Autodesk Fusion 360 part; units mm, degrees
(part 4 of 4)
  constraint vertical L5
  constraint horizontal L6
  constraint vertical L7
  constraint coincident L0.end L1.start
  constraint coincident L2.end L3.start
extrude "Extrude2" add sketch "Sketch3" along normal blind 0.36 separate body contours S0 S1 S2 S3 | S4 S5 S6 S7 | S8 S9 S10 S11 | S12 S13 S14 S15 | S16 S17 S18 S19 | S20 S21 S22 S23 | S24 S25 S26 S27 | S28 S29 S30 S31 | S32 S33 S34 S35 | S36 S37 S38 S39 | S40 S41 S42 S43 | S44 S45 S46 S47 | S48 S49 S50 S51 | S52 S53 S54 S55 | S56 S57 S58 S59 | S60 S61 S62 S63 | S64 S65 S66 S67 | S68 S69 S70 S71 | S72 S73 S74 S75 | S76 S77 S78 S79 | S80 S81 S82 S83 | S84 S85 S86 S87 | S88 S89 S90 S91 | S92 S93 S94 S95 | S96 S97 S98 S99 | S100 S101 S102 S103 | S104 S105 S106 S107 | S108 S109 S110 S111 | S112 S113 S114 S115 | S116 S117 S118 S119 | S120 S121 S122 S123 | S124 S125 S126 S127 | S128 S129 S130 S131 | S132 S133 S134 S135 | S136 S137 S138 S139 | S140 S141 S142 S143 | S144 S145 S146 S147 | S148 S149 S150 S151 | S152 S153 S154 S155 | S156 S157 S158 S159 | S160 S161 S162 S163 | S164 S165 S166 S167 | S168 S169 S170 S171 | S172 S173 S174 S175 | S176 S177 S178 S179 | S180 S181 S182 S183 | S184 S185 S186 S187 | S188 S189 S190 S191 | S192 S193 S194 S195 | S196 S197 S198 S199 | S200 S201 S202 S203 | S204 S205 S206 S207 | S208 S209 S210 S211 | S212 S213 S214 S215 | S216 S217 S218 S219 | S220 S221 S222 S223 | S224 S225 S226 S227 | S228 S229 S230 S231 | S232 S233 S234 S235 | S236 S237 S238 S239 | S240 S241 S242 S243 | S244 S245 S246 S247 | S248 S249 S250 S251 | S252 S253 S254 S255 | S256 S257 S258 S259 | S260 S261 S262 S263 | S264 S265 S266 S267 | S268 S269 S270 S271 | S272 S273 S274 S275 | S276 S277 S278 S279 | S280 S281 S282 S283 | S284 S285 S286 S287 | S288 S289 S290 S291 | S292 S293 S294 S295 | S296 S297 S298 S299 | S300 S301 S302 S303 | S304 S305 S306 S307 | S308 S309 S310 S311 | S312 S313 S314 S315 | S316 S317 S318 S319 | S320 S321 S322 S323 | S324 S325 S326 S327 | S328 S329 S330 S331 | S332 S333 S334 S335 | S336 S337 S338 S339 | S340 S341 S342 S343 | S344 S345 S346 S347 | S348 S349 S350 S351 | S352 S353 S354 S355 | S356 S357 S358 S359 | S360 S361 S362 S363 | S364 S365 S366 S367 | S368 S369 S370 S371 | S372 S373 S374 S375 | S376 S377 S378 S379 | S380 S381 S382 S383 | S384 S385 S386 S387 | S388 S389 S390 S391 | S392 S393 S394 S395 | S396 S397 S398 S399 | S400 S401 S402 S403 | S404 S405 S406 S407 | S408 S409 S410 S411 | S412 S413 S414 S415 | S416 S417 S418 S419 | S420 S421 S422 S423 | S424 S425 S426 S427 | S428 S429 S430 S431 | S432 S433 S434 S435 | S436 S437 S438 S439 | S440 S441 S442 S443 | S444 S445 S446 S447 | S448 S449 S450 S451 | S452 S453 S454 S455 | S456 S457 S458 S459 | S460 S461 S462 S463 | S464 S465 S466 S467 | S468 S469 S470 S471 | S472 S473 S474 S475 | S476 S477 S478 S479 | S480 S481 S482 S483 | S484 S485 S486 S487 | S488 S489 S490 S491 | S492 S493 S494 S495 | S496 S497 S498 S499 | S500 S501 S502 S503 | S504 S505 S506 S507 | S508 S509 S510 S511 | L0 L1 L2 L3 L4 L5 L6 L7 makes body 2
sketch "Sketch12" plane through (0, 0, 10.36) normal (0, 0, 1) x (-1, 0, 0)
  line L0 (1, 1) -> (-161, 1)
  line L1 (-161, 1) -> (-161, -81)
  line L2 (-161, -81) -> (1, -81)
  line L3 (1, -81) -> (1, 1)
  line L4 (-156, -79) -> (-4, -79)
  line L5 (-1, -76) -> (-1, -4)
  line L6 (-4, -1) -> (-156, -1)
  line L7 (-159, -4) -> (-159, -76)
  arc A0 (-1, -4) -> (-4, -1) centre (-4, -4) ccw
  arc A1 (-156, -1) -> (-159, -4) centre (-156, -4) ccw
  arc A2 (-159, -76) -> (-156, -79) centre (-156, -76) ccw
  arc A3 (-4, -79) -> (-1, -76) centre (-4, -76) ccw
  line L8 (-158, -88) -> (-2, -88)
  line L9 (8, -78) -> (8, -2)
  line L10 (-2, 8) -> (-158, 8)
  line L11 (-168, -2) -> (-168, -78)
  arc A4 (8, -2) -> (-2, 8) centre (-2, -2) ccw
  arc A5 (-2, -88) -> (8, -78) centre (-2, -78) ccw
  arc A6 (-158, 8) -> (-168, -2) centre (-158, -2) ccw
  arc A7 (-168, -78) -> (-158, -88) centre (-158, -78) ccw
  dimension "d63" = 82
  dimension "d64" = 162
  dimension "d66" = 3
  dimension "d67" = 3
  dimension "d69" = 10
  dimension "d134" = 7
  dimension "d135" = 7
  dimension "d136" = 7
  constraint horizontal L0
  constraint vertical L1
  constraint horizontal L2
  constraint vertical L3
  constraint tangent L5 A0
  constraint tangent L6 A0
  constraint tangent L6 A1
  constraint tangent L7 A1
  constraint tangent L4 A2
  constraint tangent L7 A2
  constraint equal A1 A2
  constraint tangent L4 A3
  constraint tangent L5 A3
  constraint equal A1 A3
  constraint tangent L9 A4
  constraint tangent L10 A4
  constraint tangent L8 A5
  constraint tangent L9 A5
  constraint equal A4 A5
  constraint tangent L10 A6
  constraint tangent L11 A6
  constraint equal A4 A6
  constraint tangent L8 A7
  constraint tangent L11 A7
  constraint equal A4 A7
  measures "d63" distance of L0.end L1.end
  measures "d64" distance of L0.start L0.end
  measures "d66" radius of A0
  measures "d67" radius of A1
  measures "d69" radius of A4
  measures "d134" distance of L3 L9
  measures "d135" distance of L0 L10
  measures "d136" distance of L1 L11
extrude "Extrude16" add sketch "Sketch12" along normal blind 2 separate body contours L0 L1 L2 L3 | L8 L9 L10 L11 A4 A5 A6 A7 makes body 3
sketch "Sketch13" plane through (0, 0, 10.36) normal (0, 0, -1) x (1, 0, 0)
  arc A0 (1, -76) -> (4, -79) centre (4, -76) ccw
  line L0 (1, -76) -> (1, -4)
  arc A1 (4, -1) -> (1, -4) centre (4, -4) ccw
  line L1 (4, -1) -> (156, -1)
  arc A2 (159, -4) -> (156, -1) centre (156, -4) ccw
  line L2 (159, -4) -> (159, -76)
  arc A3 (156, -79) -> (159, -76) centre (156, -76) ccw
  line L3 (156, -79) -> (4, -79)
  arc A4 (158, -88) -> (168, -78) centre (158, -78) ccw
  line L4 (168, -78) -> (168, -2)
  arc A5 (168, -2) -> (158, 8) centre (158, -2) ccw
  line L5 (158, 8) -> (2, 8)
  arc A6 (2, 8) -> (-8, -2) centre (2, -2) ccw
  line L6 (-8, -2) -> (-8, -78)
  arc A7 (-8, -78) -> (2, -88) centre (2, -78) ccw
  line L7 (2, -88) -> (158, -88)
  line L8 (-1, 1) -> (161, 1)
  line L9 (161, 1) -> (161, -81)
  line L10 (161, -81) -> (-1, -81)
  line L11 (-1, -81) -> (-1, 1)
  line L12 (-1, 1.2) -> (161, 1.2)
  dimension "d72" = -0.2
  constraint horizontal L8
  constraint vertical L9
  constraint horizontal L10
  constraint vertical L11
extrude "Extrude17" add sketch "Sketch13" along normal blind 15 separate body contours A4 L4 A5 L5 A6 L6 A7 L7 makes body 4
combine "Combine1" operation add target body 3 tool bodies 4
sketch "Sketch14" plane through (0, 0, 0) normal (0, 0, -1) x (1, 0, 0)
  line L0 (159, -78.4943) -> (151, -78.4943)
  line L1 (151, -78.4943) -> (151, -71.4943)
  line L2 (151, -71.4943) -> (159, -71.4943)
  line L3 (159, -71.4943) -> (159, -78.4943)
  line L4 (159, -68.4943) -> (151, -68.4943)
  line L5 (151, -68.4943) -> (151, -61.4943)
  line L6 (151, -61.4943) -> (159, -61.4943)
  line L7 (159, -61.4943) -> (159, -68.4943)
  line L8 (159, -58.4943) -> (151, -58.4943)
  line L9 (151, -58.4943) -> (151, -51.4943)
  line L10 (151, -51.4943) -> (159, -51.4943)
  line L11 (159, -51.4943) -> (159, -58.4943)
  line L12 (159, -48.4943) -> (151, -48.4943)
  line L13 (151, -48.4943) -> (151, -41.4943)
  line L14 (151, -41.4943) -> (159, -41.4943)
  line L15 (159, -41.4943) -> (159, -48.4943)
  line L16 (159, -38.4943) -> (151, -38.4943)
  line L17 (151, -38.4943) -> (151, -31.4943)
  line L18 (151, -31.4943) -> (159, -31.4943)
  line L19 (159, -31.4943) -> (159, -38.4943)
  line L20 (159, -28.4943) -> (151, -28.4943)
  line L21 (151, -28.4943) -> (151, -21.4943)
  line L22 (151, -21.4943) -> (159, -21.4943)
  line L23 (159, -21.4943) -> (159, -28.4943)
  line L24 (159, -18.4943) -> (151, -18.4943)
  line L25 (151, -18.4943) -> (151, -11.4943)
  line L26 (151, -11.4943) -> (159, -11.4943)
  line L27 (159, -11.4943) -> (159, -18.4943)
  line L28 (159, -8.4943) -> (151, -8.4943)
  line L29 (151, -8.4943) -> (151, -1.4943)
  line L30 (151, -1.4943) -> (159, -1.4943)
  line L31 (159, -1.4943) -> (159, -8.4943)
  line L32 (149, -78.4943) -> (141, -78.4943)
  line L33 (141, -78.4943) -> (141, -71.4943)
  line L34 (141, -71.4943) -> (149, -71.4943)
  line L35 (149, -71.4943) -> (149, -78.4943)
  line L36 (149, -68.4943) -> (141, -68.4943)
  line L37 (141, -68.4943) -> (141, -61.4943)
  line L38 (141, -61.4943) -> (149, -61.4943)
  line L39 (149, -61.4943) -> (149, -68.4943)
  line L40 (149, -58.4943) -> (141, -58.4943)
  line L41 (141, -58.4943) -> (141, -51.4943)
  line L42 (141, -51.4943) -> (149, -51.4943)
  line L43 (149, -51.4943) -> (149, -58.4943)
  line L44 (149, -48.4943) -> (141, -48.4943)
  line L45 (141, -48.4943) -> (141, -41.4943)
  line L46 (141, -41.4943) -> (149, -41.4943)
  line L47 (149, -41.4943) -> (149, -48.4943)
  line L48 (149, -38.4943) -> (141, -38.4943)
  line L49 (141, -38.4943) -> (141, -31.4943)
  line L50 (141, -31.4943) -> (149, -31.4943)
  line L51 (149, -31.4943) -> (149, -38.4943)
  line L52 (149, -28.4943) -> (141, -28.4943)
  line L53 (141, -28.4943) -> (141, -21.4943)
  line L54 (141, -21.4943) -> (149, -21.4943)
  line L55 (149, -21.4943) -> (149, -28.4943)
  line L56 (149, -18.4943) -> (141, -18.4943)
  line L57 (141, -18.4943) -> (141, -11.4943)
  line L58 (141, -11.4943) -> (149, -11.4943)
  line L59 (149, -11.4943) -> (149, -18.4943)
  line L60 (149, -8.4943) -> (141, -8.4943)
  line L61 (141, -8.4943) -> (141, -1.4943)
  line L62 (141, -1.4943) -> (149, -1.4943)
  line L63 (149, -1.4943) -> (149, -8.4943)
  line L64 (139, -78.4943) -> (131, -78.4943)
  line L65 (131, -78.4943) -> (131, -71.4943)
  line L66 (131, -71.4943) -> (139, -71.4943)
  line L67 (139, -71.4943) -> (139, -78.4943)
  line L68 (139, -68.4943) -> (131, -68.4943)
  line L69 (131, -68.4943) -> (131, -61.4943)
  line L70 (131, -61.4943) -> (139, -61.4943)
  line L71 (139, -61.4943) -> (139, -68.4943)
  line L72 (139, -58.4943) -> (131, -58.4943)
  line L73 (131, -58.4943) -> (131, -51.4943)
  line L74 (131, -51.4943) -> (139, -51.4943)
  line L75 (139, -51.4943) -> (139, -58.4943)
  line L76 (139, -48.4943) -> (131, -48.4943)
  line L77 (131, -48.4943) -> (131, -41.4943)
  line L78 (131, -41.4943) -> (139, -41.4943)
  line L79 (139, -41.4943) -> (139, -48.4943)
  line L80 (139, -38.4943) -> (131, -38.4943)
  line L81 (131, -38.4943) -> (131, -31.4943)
  line L82 (131, -31.4943) -> (139, -31.4943)
  line L83 (139, -31.4943) -> (139, -38.4943)
  line L84 (139, -28.4943) -> (131, -28.4943)
  line L85 (131, -28.4943) -> (131, -21.4943)
  line L86 (131, -21.4943) -> (139, -21.4943)
  line L87 (139, -21.4943) -> (139, -28.4943)
  line L88 (139, -18.4943) -> (131, -18.4943)
  line L89 (131, -18.4943) -> (131, -11.4943)
  line L90 (131, -11.4943) -> (139, -11.4943)
  line L91 (139, -11.4943) -> (139, -18.4943)
  line L92 (139, -8.4943) -> (131, -8.4943)
  line L93 (131, -8.4943) -> (131, -1.4943)
  line L94 (131, -1.4943) -> (139, -1.4943)
  line L95 (139, -1.4943) -> (139, -8.4943)
  line L96 (129, -78.4943) -> (121, -78.4943)
  line L97 (121, -78.4943) -> (121, -71.4943)
  line L98 (121, -71.4943) -> (129, -71.4943)
  line L99 (129, -71.4943) -> (129, -78.4943)
  line L100 (129, -68.4943) -> (121, -68.4943)
  line L101 (121, -68.4943) -> (121, -61.4943)
  line L102 (121, -61.4943) -> (129, -61.4943)
  line L103 (129, -61.4943) -> (129, -68.4943)
  line L104 (129, -58.4943) -> (121, -58.4943)
  line L105 (121, -58.4943) -> (121, -51.4943)
  line L106 (121, -51.4943) -> (129, -51.4943)
  line L107 (129, -51.4943) -> (129, -58.4943)
  line L108 (129, -48.4943) -> (121, -48.4943)
  line L109 (121, -48.4943) -> (121, -41.4943)
  line L110 (121, -41.4943) -> (129, -41.4943)
  line L111 (129, -41.4943) -> (129, -48.4943)
  line L112 (129, -38.4943) -> (121, -38.4943)
  line L113 (121, -38.4943) -> (121, -31.4943)
  line L114 (121, -31.4943) -> (129, -31.4943)
  line L115 (129, -31.4943) -> (129, -38.4943)
  line L116 (129, -28.4943) -> (121, -28.4943)
  line L117 (121, -28.4943) -> (121, -21.4943)
  line L118 (121, -21.4943) -> (129, -21.4943)
  line L119 (129, -21.4943) -> (129, -28.4943)
  line L120 (129, -18.4943) -> (121, -18.4943)
  line L121 (121, -18.4943) -> (121, -11.4943)
  line L122 (121, -11.4943) -> (129, -11.4943)
  line L123 (129, -11.4943) -> (129, -18.4943)
  line L124 (129, -8.4943) -> (121, -8.4943)
  line L125 (121, -8.4943) -> (121, -1.4943)
  line L126 (121, -1.4943) -> (129, -1.4943)
  line L127 (129, -1.4943) -> (129, -8.4943)
  line L128 (119, -78.4943) -> (111, -78.4943)
  line L129 (111, -78.4943) -> (111, -71.4943)
  line L130 (111, -71.4943) -> (119, -71.4943)
  line L131 (119, -71.4943) -> (119, -78.4943)
  line L132 (119, -68.4943) -> (111, -68.4943)
  line L133 (111, -68.4943) -> (111, -61.4943)
  line L134 (111, -61.4943) -> (119, -61.4943)
  line L135 (119, -61.4943) -> (119, -68.4943)
  line L136 (119, -58.4943) -> (111, -58.4943)
  line L137 (111, -58.4943) -> (111, -51.4943)
  line L138 (111, -51.4943) -> (119, -51.4943)
  line L139 (119, -51.4943) -> (119, -58.4943)
  line L140 (119, -48.4943) -> (111, -48.4943)
  line L141 (111, -48.4943) -> (111, -41.4943)
  line L142 (111, -41.4943) -> (119, -41.4943)
  line L143 (119, -41.4943) -> (119, -48.4943)
  line L144 (119, -38.4943) -> (111, -38.4943)
  line L145 (111, -38.4943) -> (111, -31.4943)
  line L146 (111, -31.4943) -> (119, -31.4943)
  line L147 (119, -31.4943) -> (119, -38.4943)
  line L148 (119, -28.4943) -> (111, -28.4943)
  line L149 (111, -28.4943) -> (111, -21.4943)
  line L150 (111, -21.4943) -> (119, -21.4943)
  line L151 (119, -21.4943) -> (119, -28.4943)
  line L152 (119, -18.4943) -> (111, -18.4943)
  line L153 (111, -18.4943) -> (111, -11.4943)
  line L154 (111, -11.4943) -> (119, -11.4943)
  line L155 (119, -11.4943) -> (119, -18.4943)
  line L156 (119, -8.4943) -> (111, -8.4943)
  line L157 (111, -8.4943) -> (111, -1.4943)
  line L158 (111, -1.4943) -> (119, -1.4943)
  line L159 (119, -1.4943) -> (119, -8.4943)
  line L160 (109, -78.4943) -> (101, -78.4943)
  line L161 (101, -78.4943) -> (101, -71.4943)
  line L162 (101, -71.4943) -> (109, -71.4943)
  line L163 (109, -71.4943) -> (109, -78.4943)
  line L164 (109, -68.4943) -> (101, -68.4943)
  line L165 (101, -68.4943) -> (101, -61.4943)
  line L166 (101, -61.4943) -> (109, -61.4943)
  line L167 (109, -61.4943) -> (109, -68.4943)
  line L168 (109, -58.4943) -> (101, -58.4943)
  line L169 (101, -58.4943) -> (101, -51.4943)
  line L170 (101, -51.4943) -> (109, -51.4943)
  line L171 (109, -51.4943) -> (109, -58.4943)
  line L172 (109, -48.4943) -> (101, -48.4943)
  line L173 (101, -48.4943) -> (101, -41.4943)
  line L174 (101, -41.4943) -> (109, -41.4943)
  line L175 (109, -41.4943) -> (109, -48.4943)
  line L176 (109, -38.4943) -> (101, -38.4943)
  line L177 (101, -38.4943) -> (101, -31.4943)
  line L178 (101, -31.4943) -> (109, -31.4943)
  line L179 (109, -31.4943) -> (109, -38.4943)
  line L180 (109, -28.4943) -> (101, -28.4943)
  line L181 (101, -28.4943) -> (101, -21.4943)
  line L182 (101, -21.4943) -> (109, -21.4943)
  line L183 (109, -21.4943) -> (109, -28.4943)
  line L184 (109, -18.4943) -> (101, -18.4943)
  line L185 (101, -18.4943) -> (101, -11.4943)
  line L186 (101, -11.4943) -> (109, -11.4943)
  line L187 (109, -11.4943) -> (109, -18.4943)
  line L188 (109, -8.4943) -> (101, -8.4943)
  line L189 (101, -8.4943) -> (101, -1.4943)
  line L190 (101, -1.4943) -> (109, -1.4943)
  line L191 (109, -1.4943) -> (109, -8.4943)
  line L192 (99, -78.4943) -> (91, -78.4943)
  line L193 (91, -78.4943) -> (91, -71.4943)
  line L194 (91, -71.4943) -> (99, -71.4943)
  line L195 (99, -71.4943) -> (99, -78.4943)
  line L196 (99, -68.4943) -> (91, -68.4943)
  line L197 (91, -68.4943) -> (91, -61.4943)
  line L198 (91, -61.4943) -> (99, -61.4943)
  line L199 (99, -61.4943) -> (99, -68.4943)
  line L200 (99, -58.4943) -> (91, -58.4943)
  line L201 (91, -58.4943) -> (91, -51.4943)
  line L202 (91, -51.4943) -> (99, -51.4943)
  line L203 (99, -51.4943) -> (99, -58.4943)
  line L204 (99, -48.4943) -> (91, -48.4943)
  line L205 (91, -48.4943) -> (91, -41.4943)
  line L206 (91, -41.4943) -> (99, -41.4943)
  line L207 (99, -41.4943) -> (99, -48.4943)
  line L208 (99, -38.4943) -> (91, -38.4943)
  line L209 (91, -38.4943) -> (91, -31.4943)
  line L210 (91, -31.4943) -> (99, -31.4943)
  line L211 (99, -31.4943) -> (99, -38.4943)
  line L212 (99, -28.4943) -> (91, -28.4943)
  line L213 (91, -28.4943) -> (91, -21.4943)
  line L214 (91, -21.4943) -> (99, -21.4943)
  line L215 (99, -21.4943) -> (99, -28.4943)
  line L216 (99, -18.4943) -> (91, -18.4943)
  line L217 (91, -18.4943) -> (91, -11.4943)
  line L218 (91, -11.4943) -> (99, -11.4943)
  line L219 (99, -11.4943) -> (99, -18.4943)
  line L220 (99, -8.4943) -> (91, -8.4943)
  line L221 (91, -8.4943) -> (91, -1.4943)
  line L222 (91, -1.4943) -> (99, -1.4943)
  line L223 (99, -1.4943) -> (99, -8.4943)
  line L224 (89, -78.4943) -> (81, -78.4943)
  line L225 (81, -78.4943) -> (81, -71.4943)
  line L226 (81, -71.4943) -> (89, -71.4943)
  line L227 (89, -71.4943) -> (89, -78.4943)
  line L228 (89, -68.4943) -> (81, -68.4943)
  line L229 (81, -68.4943) -> (81, -61.4943)
  line L230 (81, -61.4943) -> (89, -61.4943)
  line L231 (89, -61.4943) -> (89, -68.4943)
  line L232 (89, -58.4943) -> (81, -58.4943)
  line L233 (81, -58.4943) -> (81, -51.4943)
  line L234 (81, -51.4943) -> (89, -51.4943)
  line L235 (89, -51.4943) -> (89, -58.4943)
  line L236 (89, -48.4943) -> (81, -48.4943)
  line L237 (81, -48.4943) -> (81, -41.4943)
  line L238 (81, -41.4943) -> (89, -41.4943)
  line L239 (89, -41.4943) -> (89, -48.4943)
  line L240 (89, -38.4943) -> (81, -38.4943)
  line L241 (81, -38.4943) -> (81, -31.4943)
  line L242 (81, -31.4943) -> (89, -31.4943)
  line L243 (89, -31.4943) -> (89, -38.4943)
  line L244 (89, -28.4943) -> (81, -28.4943)
  line L245 (81, -28.4943) -> (81, -21.4943)
  line L246 (81, -21.4943) -> (89, -21.4943)
  line L247 (89, -21.4943) -> (89, -28.4943)
  line L248 (89, -18.4943) -> (81, -18.4943)
  line L249 (81, -18.4943) -> (81, -11.4943)
  line L250 (81, -11.4943) -> (89, -11.4943)
  line L251 (89, -11.4943) -> (89, -18.4943)
  line L252 (89, -8.4943) -> (81, -8.4943)
  line L253 (81, -8.4943) -> (81, -1.4943)
  line L254 (81, -1.4943) -> (89, -1.4943)
  line L255 (89, -1.4943) -> (89, -8.4943)
  line L256 (79, -78.4943) -> (71, -78.4943)
  line L257 (71, -78.4943) -> (71, -71.4943)
  line L258 (71, -71.4943) -> (79, -71.4943)
  line L259 (79, -71.4943) -> (79, -78.4943)
  line L260 (79, -68.4943) -> (71, -68.4943)
  line L261 (71, -68.4943) -> (71, -61.4943)
  line L262 (71, -61.4943) -> (79, -61.4943)
  line L263 (79, -61.4943) -> (79, -68.4943)
  line L264 (79, -58.4943) -> (71, -58.4943)
  line L265 (71, -58.4943) -> (71, -51.4943)
  line L266 (71, -51.4943) -> (79, -51.4943)
  line L267 (79, -51.4943) -> (79, -58.4943)
  line L268 (79, -48.4943) -> (71, -48.4943)
  line L269 (71, -48.4943) -> (71, -41.4943)
  line L270 (71, -41.4943) -> (79, -41.4943)
  line L271 (79, -41.4943) -> (79, -48.4943)
  line L272 (79, -38.4943) -> (71, -38.4943)
  line L273 (71, -38.4943) -> (71, -31.4943)
  line L274 (71, -31.4943) -> (79, -31.4943)
  line L275 (79, -31.4943) -> (79, -38.4943)
  line L276 (79, -28.4943) -> (71, -28.4943)
  line L277 (71, -28.4943) -> (71, -21.4943)
  line L278 (71, -21.4943) -> (79, -21.4943)
  line L279 (79, -21.4943) -> (79, -28.4943)
  line L280 (79, -18.4943) -> (71, -18.4943)
  line L281 (71, -18.4943) -> (71, -11.4943)
  line L282 (71, -11.4943) -> (79, -11.4943)
  line L283 (79, -11.4943) -> (79, -18.4943)
  line L284 (79, -8.4943) -> (71, -8.4943)
  line L285 (71, -8.4943) -> (71, -1.4943)
  line L286 (71, -1.4943) -> (79, -1.4943)
  line L287 (79, -1.4943) -> (79, -8.4943)
  line L288 (69, -78.4943) -> (61, -78.4943)
  line L289 (61, -78.4943) -> (61, -71.4943)
  line L290 (61, -71.4943) -> (69, -71.4943)
  line L291 (69, -71.4943) -> (69, -78.4943)
  line L292 (69, -68.4943) -> (61, -68.4943)
  line L293 (61, -68.4943) -> (61, -61.4943)
  line L294 (61, -61.4943) -> (69, -61.4943)
  line L295 (69, -61.4943) -> (69, -68.4943)
  line L296 (69, -58.4943) -> (61, -58.4943)
  line L297 (61, -58.4943) -> (61, -51.4943)
  line L298 (61, -51.4943) -> (69, -51.4943)
  line L299 (69, -51.4943) -> (69, -58.4943)
  line L300 (69, -48.4943) -> (61, -48.4943)
  line L301 (61, -48.4943) -> (61, -41.4943)
  line L302 (61, -41.4943) -> (69, -41.4943)
  line L303 (69, -41.4943) -> (69, -48.4943)
  line L304 (69, -38.4943) -> (61, -38.4943)
  line L305 (61, -38.4943) -> (61, -31.4943)
  line L306 (61, -31.4943) -> (69, -31.4943)
  line L307 (69, -31.4943) -> (69, -38.4943)
  line L308 (69, -28.4943) -> (61, -28.4943)
  line L309 (61, -28.4943) -> (61, -21.4943)
  line L310 (61, -21.4943) -> (69, -21.4943)
  line L311 (69, -21.4943) -> (69, -28.4943)
  line L312 (69, -18.4943) -> (61, -18.4943)
  line L313 (61, -18.4943) -> (61, -11.4943)
  line L314 (61, -11.4943) -> (69, -11.4943)
  line L315 (69, -11.4943) -> (69, -18.4943)
  line L316 (69, -8.4943) -> (61, -8.4943)
  line L317 (61, -8.4943) -> (61, -1.4943)
  line L318 (61, -1.4943) -> (69, -1.4943)
  line L319 (69, -1.4943) -> (69, -8.4943)
  line L320 (59, -78.4943) -> (51, -78.4943)
  line L321 (51, -78.4943) -> (51, -71.4943)
  line L322 (51, -71.4943) -> (59, -71.4943)
  line L323 (59, -71.4943) -> (59, -78.4943)
  line L324 (59, -68.4943) -> (51, -68.4943)
  line L325 (51, -68.4943) -> (51, -61.4943)
  line L326 (51, -61.4943) -> (59, -61.4943)
  line L327 (59, -61.4943) -> (59, -68.4943)
  line L328 (59, -58.4943) -> (51, -58.4943)
  line L329 (51, -58.4943) -> (51, -51.4943)
  line L330 (51, -51.4943) -> (59, -51.4943)
  line L331 (59, -51.4943) -> (59, -58.4943)
  line L332 (59, -48.4943) -> (51, -48.4943)
  line L333 (51, -48.4943) -> (51, -41.4943)
  line L334 (51, -41.4943) -> (59, -41.4943)
  line L335 (59, -41.4943) -> (59, -48.4943)
  line L336 (59, -38.4943) -> (51, -38.4943)
  line L337 (51, -38.4943) -> (51, -31.4943)
  line L338 (51, -31.4943) -> (59, -31.4943)
  line L339 (59, -31.4943) -> (59, -38.4943)
  line L340 (59, -28.4943) -> (51, -28.4943)
  line L341 (51, -28.4943) -> (51, -21.4943)
  line L342 (51, -21.4943) -> (59, -21.4943)
  line L343 (59, -21.4943) -> (59, -28.4943)
  line L344 (59, -18.4943) -> (51, -18.4943)
  line L345 (51, -18.4943) -> (51, -11.4943)
  line L346 (51, -11.4943) -> (59, -11.4943)
  line L347 (59, -11.4943) -> (59, -18.4943)
  line L348 (59, -8.4943) -> (51, -8.4943)
  line L349 (51, -8.4943) -> (51, -1.4943)
  line L350 (51, -1.4943) -> (59, -1.4943)
  line L351 (59, -1.4943) -> (59, -8.4943)
  line L352 (49, -78.4943) -> (41, -78.4943)
  line L353 (41, -78.4943) -> (41, -71.4943)
  line L354 (41, -71.4943) -> (49, -71.4943)
  line L355 (49, -71.4943) -> (49, -78.4943)
  line L356 (49, -68.4943) -> (41, -68.4943)
  line L357 (41, -68.4943) -> (41, -61.4943)
  line L358 (41, -61.4943) -> (49, -61.4943)
  line L359 (49, -61.4943) -> (49, -68.4943)
  line L360 (49, -58.4943) -> (41, -58.4943)
  line L361 (41, -58.4943) -> (41, -51.4943)
  line L362 (41, -51.4943) -> (49, -51.4943)
  line L363 (49, -51.4943) -> (49, -58.4943)
  line L364 (49, -48.4943) -> (41, -48.4943)
  line L365 (41, -48.4943) -> (41, -41.4943)
  line L366 (41, -41.4943) -> (49, -41.4943)
  line L367 (49, -41.4943) -> (49, -48.4943)
  line L368 (49, -38.4943) -> (41, -38.4943)
  line L369 (41, -38.4943) -> (41, -31.4943)
  line L370 (41, -31.4943) -> (49, -31.4943)
  line L371 (49, -31.4943) -> (49, -38.4943)
  line L372 (49, -28.4943) -> (41, -28.4943)
  line L373 (41, -28.4943) -> (41, -21.4943)
  line L374 (41, -21.4943) -> (49, -21.4943)
  line L375 (49, -21.4943) -> (49, -28.4943)
  line L376 (49, -18.4943) -> (41, -18.4943)
  line L377 (41, -18.4943) -> (41, -11.4943)
  line L378 (41, -11.4943) -> (49, -11.4943)
  line L379 (49, -11.4943) -> (49, -18.4943)
  line L380 (49, -8.4943) -> (41, -8.4943)
  line L381 (41, -8.4943) -> (41, -1.4943)
  line L382 (41, -1.4943) -> (49, -1.4943)
  line L383 (49, -1.4943) -> (49, -8.4943)
  line L384 (39, -78.4943) -> (31, -78.4943)
  line L385 (31, -78.4943) -> (31, -71.4943)
  line L386 (31, -71.4943) -> (39, -71.4943)
  line L387 (39, -71.4943) -> (39, -78.4943)
  line L388 (39, -68.4943) -> (31, -68.4943)
  line L389 (31, -68.4943) -> (31, -61.4943)
  line L390 (31, -61.4943) -> (39, -61.4943)
  line L391 (39, -61.4943) -> (39, -68.4943)
  line L392 (39, -58.4943) -> (31, -58.4943)
  line L393 (31, -58.4943) -> (31, -51.4943)
  line L394 (31, -51.4943) -> (39, -51.4943)
  line L395 (39, -51.4943) -> (39, -58.4943)
  line L396 (39, -48.4943) -> (31, -48.4943)
  line L397 (31, -48.4943) -> (31, -41.4943)
  line L398 (31, -41.4943) -> (39, -41.4943)
  line L399 (39, -41.4943) -> (39, -48.4943)
  line L400 (39, -38.4943) -> (31, -38.4943)
  line L401 (31, -38.4943) -> (31, -31.4943)
  line L402 (31, -31.4943) -> (39, -31.4943)
  line L403 (39, -31.4943) -> (39, -38.4943)
  line L404 (39, -28.4943) -> (31, -28.4943)
  line L405 (31, -28.4943) -> (31, -21.4943)
  line L406 (31, -21.4943) -> (39, -21.4943)
  line L407 (39, -21.4943) -> (39, -28.4943)
  line L408 (39, -18.4943) -> (31, -18.4943)
  line L409 (31, -18.4943) -> (31, -11.4943)
  line L410 (31, -11.4943) -> (39, -11.4943)
  line L411 (39, -11.4943) -> (39, -18.4943)
  line L412 (39, -8.4943) -> (31, -8.4943)
  line L413 (31, -8.4943) -> (31, -1.4943)
  line L414 (31, -1.4943) -> (39, -1.4943)
  line L415 (39, -1.4943) -> (39, -8.4943)
  line L416 (29, -78.4943) -> (21, -78.4943)
  line L417 (21, -78.4943) -> (21, -71.4943)
  line L418 (21, -71.4943) -> (29, -71.4943)
  line L419 (29, -71.4943) -> (29, -78.4943)
  line L420 (29, -68.4943) -> (21, -68.4943)
  line L421 (21, -68.4943) -> (21, -61.4943)
  line L422 (21, -61.4943) -> (29, -61.4943)
  line L423 (29, -61.4943) -> (29, -68.4943)
  line L424 (29, -58.4943) -> (21, -58.4943)
  line L425 (21, -58.4943) -> (21, -51.4943)
  line L426 (21, -51.4943) -> (29, -51.4943)
  line L427 (29, -51.4943) -> (29, -58.4943)
  line L428 (29, -48.4943) -> (21, -48.4943)
  line L429 (21, -48.4943) -> (21, -41.4943)
  line L430 (21, -41.4943) -> (29, -41.4943)
  line L431 (29, -41.4943) -> (29, -48.4943)
  line L432 (29, -38.4943) -> (21, -38.4943)
  line L433 (21, -38.4943) -> (21, -31.4943)
  line L434 (21, -31.4943) -> (29, -31.4943)
  line L435 (29, -31.4943) -> (29, -38.4943)
  line L436 (29, -28.4943) -> (21, -28.4943)
  line L437 (21, -28.4943) -> (21, -21.4943)
  line L438 (21, -21.4943) -> (29, -21.4943)
  line L439 (29, -21.4943) -> (29, -28.4943)
  line L440 (29, -18.4943) -> (21, -18.4943)
  line L441 (21, -18.4943) -> (21, -11.4943)
  line L442 (21, -11.4943) -> (29, -11.4943)
  line L443 (29, -11.4943) -> (29, -18.4943)
  line L444 (29, -8.4943) -> (21, -8.4943)
  line L445 (21, -8.4943) -> (21, -1.4943)
  line L446 (21, -1.4943) -> (29, -1.4943)
  line L447 (29, -1.4943) -> (29, -8.4943)
  line L448 (19, -78.4943) -> (11, -78.4943)
  line L449 (11, -78.4943) -> (11, -71.4943)
  line L450 (11, -71.4943) -> (19, -71.4943)
  line L451 (19, -71.4943) -> (19, -78.4943)
  line L452 (19, -68.4943) -> (11, -68.4943)
  line L453 (11, -68.4943) -> (11, -61.4943)
  line L454 (11, -61.4943) -> (19, -61.4943)
  line L455 (19, -61.4943) -> (19, -68.4943)
  line L456 (19, -58.4943) -> (11, -58.4943)
  line L457 (11, -58.4943) -> (11, -51.4943)
  line L458 (11, -51.4943) -> (19, -51.4943)
  line L459 (19, -51.4943) -> (19, -58.4943)
  line L460 (19, -48.4943) -> (11, -48.4943)
  line L461 (11, -48.4943) -> (11, -41.4943)
  line L462 (11, -41.4943) -> (19, -41.4943)
  line L463 (19, -41.4943) -> (19, -48.4943)
  line L464 (19, -38.4943) -> (11, -38.4943)
  line L465 (11, -38.4943) -> (11, -31.4943)
  line L466 (11, -31.4943) -> (19, -31.4943)
  line L467 (19, -31.4943) -> (19, -38.4943)
  line L468 (19, -28.4943) -> (11, -28.4943)
  line L469 (11, -28.4943) -> (11, -21.4943)
  line L470 (11, -21.4943) -> (19, -21.4943)
  line L471 (19, -21.4943) -> (19, -28.4943)
  line L472 (19, -18.4943) -> (11, -18.4943)
  line L473 (11, -18.4943) -> (11, -11.4943)
  line L474 (11, -11.4943) -> (19, -11.4943)
  line L475 (19, -11.4943) -> (19, -18.4943)
  line L476 (19, -8.4943) -> (11, -8.4943)
  line L477 (11, -8.4943) -> (11, -1.4943)
  line L478 (11, -1.4943) -> (19, -1.4943)
  line L479 (19, -1.4943) -> (19, -8.4943)
  line L480 (9, -78.4943) -> (1, -78.4943)
  line L481 (1, -78.4943) -> (1, -71.4943)
  line L482 (1, -71.4943) -> (9, -71.4943)
  line L483 (9, -71.4943) -> (9, -78.4943)
  line L484 (9, -68.4943) -> (1, -68.4943)
  line L485 (1, -68.4943) -> (1, -61.4943)
  line L486 (1, -61.4943) -> (9, -61.4943)
  line L487 (9, -61.4943) -> (9, -68.4943)
  line L488 (9, -58.4943) -> (1, -58.4943)
  line L489 (1, -58.4943) -> (1, -51.4943)
  line L490 (1, -51.4943) -> (9, -51.4943)
  line L491 (9, -51.4943) -> (9, -58.4943)
  line L492 (9, -48.4943) -> (1, -48.4943)
  line L493 (1, -48.4943) -> (1, -41.4943)
  line L494 (1, -41.4943) -> (9, -41.4943)
  line L495 (9, -41.4943) -> (9, -48.4943)
  line L496 (9, -38.4943) -> (1, -38.4943)
  line L497 (1, -38.4943) -> (1, -31.4943)
  line L498 (1, -31.4943) -> (9, -31.4943)
  line L499 (9, -31.4943) -> (9, -38.4943)
  line L500 (9, -28.4943) -> (1, -28.4943)
  line L501 (1, -28.4943) -> (1, -21.4943)
  line L502 (1, -21.4943) -> (9, -21.4943)
  line L503 (9, -21.4943) -> (9, -28.4943)
  line L504 (9, -18.4943) -> (1, -18.4943)
  line L505 (1, -18.4943) -> (1, -11.4943)
  line L506 (1, -11.4943) -> (9, -11.4943)
  line L507 (9, -11.4943) -> (9, -18.4943)
  line L508 (9, -8.4943) -> (1, -8.4943)
  line L509 (1, -8.4943) -> (1, -1.4943)
  line L510 (1, -1.4943) -> (9, -1.4943)
  line L511 (9, -1.4943) -> (9, -8.4943)
  line L512 (161, 1) -> (-1, 1)
  line L513 (-1, 1) -> (-1, -81)
  line L514 (-1, -81) -> (161, -81)
  line L515 (161, -81) -> (161, 1)
  line L516 (-1, 1) -> (161, 1)
  line L517 (161, 1) -> (161, -81)
  line L518 (161, -81) -> (-1, -81)
  line L519 (-1, -81) -> (-1, 1)
  line L520 (-0.5, -81) -> (-0.5, 0.5)
  line L521 (-0.5, 0.5) -> (161, 0.5)
  line L522 (-1, 1) -> (-1, -19)
  line L523 (-1, -19) -> (3, -19)
  line L524 (-1, -81) -> (-1, -61)
  line L525 (-1, -61) -> (3, -61)
  line L526 (6, -71) -> (6, -64)
  line L527 (6, -16) -> (6, -9)
  line L528 (75.1065, -9) -> (75.1065, -74)
  line L529 (79, -74) -> (80.1065, -74)
  line L530 (80.1065, -6) -> (79, -6)
  line L531 (75.1065, -6) -> (75.1065, -71)
  line L532 (83.1065, -37.5) -> (153.9065, -37.5)
  line L533 (153.9065, -42.5) -> (83.1065, -42.5)
  line L534 (153.9065, -37.5) -> (151, -37.5)
  line L535 (151, -42.5) -> (153.9065, -42.5)
  line L536 (80.1065, -71) -> (80.1065, -45.5)
  line L537 (80.1065, -34.5) -> (80.1065, -9)
  line L538 (154, -9) -> (154, -34.5)
  line L539 (154, -45.5) -> (154, -71)
  line L540 (151, -74) -> (83.1065, -74)
  line L541 (72.1065, -74) -> (9, -74)
  line L542 (9, -6) -> (72.1065, -6)
  line L543 (83.1065, -6) -> (151, -6)
  arc A0 (75.1065, -9) -> (72.1065, -6) centre (72.1065, -9) ccw
  arc A1 (83.1065, -6) -> (80.1065, -9) centre (83.1065, -9) ccw
  arc A2 (80.1065, -34.5) -> (83.1065, -37.5) centre (83.1065, -34.5) ccw
  arc A3 (83.1065, -42.5) -> (80.1065, -45.5) centre (83.1065, -45.5) ccw
  arc A4 (151, -37.5) -> (154, -34.5) centre (151, -34.5) ccw
  arc A5 (154, -9) -> (151, -6) centre (151, -9) ccw
  arc A6 (154, -45.5) -> (151, -42.5) centre (151, -45.5) ccw
  arc A7 (80.1065, -71) -> (83.1065, -74) centre (83.1065, -71) ccw
  arc A8 (151, -74) -> (154, -71) centre (151, -71) ccw
  arc A9 (72.1065, -74) -> (75.1065, -71) centre (72.1065, -71) ccw
  arc A10 (6, -71) -> (9, -74) centre (9, -71) ccw
  arc A11 (6, -64) -> (3, -61) centre (3, -64) ccw
  arc A12 (3, -19) -> (6, -16) centre (3, -16) ccw
  arc A13 (9, -6) -> (6, -9) centre (9, -9) ccw
  point P0 (80.1065, -37.5)
  point P1 (80.1065, -42.5)
  dimension "d75" = 0.5
  dimension "d77" = 20
  dimension "d78" = 5
  dimension "d80" = 73.8
  dimension "d81" = 5
  dimension "d82" = 3
  constraint horizontal L516
  constraint vertical L517
  constraint horizontal L518
  constraint vertical L519
  constraint coincident L514.end L515.start
  constraint coincident L512.end L513.start
  constraint perpendicular L512 L522
  constraint perpendicular L523 L526
  constraint coincident L513 L524.end
  constraint perpendicular L525 L526
  constraint collinear L526 L527
  constraint coincident L528.end L540
  constraint perpendicular L528 L540
  constraint horizontal L529
  constraint vertical L536
  constraint horizontal L530
  constraint vertical L531
  constraint coincident L530.start L542
  constraint horizontal L532
  constraint horizontal L533
  constraint horizontal L534
  constraint horizontal L535
  constraint collinear L536 L537
  constraint collinear L538 L539
  constraint coincident L259 L529.start
  constraint collinear L540 L541
  constraint coincident L287 L530.end
  constraint collinear L542 L543
  constraint tangent L528 A0
  constraint tangent L542 A0
  constraint coincident L530.start L537
  constraint tangent L543 A1
  constraint tangent L537 A1
  constraint equal A0 A1
  constraint coincident P0 L532
  constraint coincident P0 L537
  constraint tangent L532 A2
  constraint tangent L537 A2
  constraint equal A0 A2
  constraint coincident P1 L533
  constraint coincident P1 L536
  constraint tangent L533 A3
  constraint tangent L536 A3
  constraint equal A0 A3
  constraint tangent L534 A4
  constraint tangent L538 A4
  constraint equal A0 A4
  constraint tangent L538 A5
  constraint tangent L543 A5
  constraint equal A0 A5
  constraint tangent L535 A6
  constraint tangent L539 A6
  constraint equal A0 A6
  constraint coincident L529.start L540
  constraint coincident L529.end L536
  constraint tangent L540 A7
  constraint tangent L536 A7
  constraint equal A0 A7
  constraint tangent L539 A8
  constraint tangent L540 A8
  constraint equal A0 A8
  constraint coincident L528.end L531
  constraint tangent L541 A9
  constraint tangent L531 A9
  constraint equal A0 A9
  constraint tangent L526 A10
  constraint tangent L541 A10
  constraint equal A0 A10
  constraint tangent L525 A11
  constraint tangent L526 A11
  constraint equal A0 A11
  constraint tangent L523 A12
  constraint tangent L527 A12
  constraint equal A0 A12
  constraint tangent L527 A13
  constraint tangent L542 A13
  constraint equal A0 A13
  measures "d77" distance of L512.end L522.end
  measures "d78" distance of L528.end L529.end
  measures "d80" distance of P0 L532.end
  measures "d81" distance of P0 P1
  measures "d82" radius of A0
extrude "Extrude18" add sketch "Sketch14" along normal blind 4.64 separate body contours L0 L1 L2 L3 A8 | L32 L33 L35 L540 | L4 L6 L7 L539 | L64 L65 L67 L540 | L8 L10 L11 L539 | L96 L97 L99 L540 | L12 L13 L14 L15 L539 A6 | L128 L129 L131 L540 | L160 L161 L163 L540 | L45 L46 L47 L533 | L192 L193 L195 L540 | L77 L78 L79 L533 | L224 L225 L227 L540 A7 | L109 L110 L111 L533 | L141 L142 L143 L533 | L173 L174 L175 L533 | L237 L238 L239 L533 A3 | L205 L206 L207 L533 | L16 L17 L18 L19 L538 A4 | L48 L49 L51 L532 | L20 L22 L23 L538 | L80 L81 L83 L532 | L24 L26 L27 L538 | L112 L113 L115 L532 | L28 L29 L30 L31 A5 | L144 L145 L147 L532 | L61 L62 L63 L543 | L176 L177 L179 L532 | L93 L94 L95 L543 | L208 L209 L211 L532 | L125 L126 L127 L543 | L240 L241 L243 L532 A2 | L157 L158 L159 L543 | L189 L190 L191 L543 | L253 L254 L255 L543 A1 | L221 L222 L223 L543 | L256 L257 L258 L259 L260 L262 L263 L264 L266 L267 L268 L270 L271 L272 L274 L275 L276 L278 L279 L280 L282 L283 L284 L285 L286 L287 L288 L289 L291 L317 L318 L319 L320 L321 L323 L349 L350 L351 L352 L353 L355 L381 L382 L383 L384 L385 L387 L413 L414 L415 L416 L417 L419 L445 L446 L447 L448 L449 L451 L477 L478 L479 L480 L481 L482 L483 L484 L485 L486 L504 L505 L506 L508 L509 L510 L511 L514 L515 L517 L518 L520 L521 L523 L525 L526 L527 L528 L531 L541 L542 A10 A11 A12 A13 | L256 L257 L258 L259 L541 A9 | L288 L289 L291 L541 | L320 L321 L323 L541 | L260 L262 L263 L528 L531 | L352 L353 L355 L541 | L264 L266 L267 L528 L531 | L384 L385 L387 L541 | L268 L270 L271 L528 L531 | L416 L417 L419 L541 | L272 L274 L275 L528 L531 | L448 L449 L451 L541 | L276 L278 L279 L528 L531 | L480 L481 L482 L483 A10 | L280 L282 L283 L528 L531 | L484 L485 L486 L526 A11 | L284 L285 L286 L287 L542 A0 | L317 L318 L319 L542 | L349 L350 L351 L542 | L504 L505 L506 L527 A12 | L381 L382 L383 L542 | L413 L414 L415 L542 | L508 L509 L510 L511 A13 | L445 L446 L447 L542 | L477 L478 L479 L542 makes body 5
sketch "Sketch15" plane through (0, 0, -4.64) normal (0, 0, -1) x (1, 0, 0)
  line L0 (161, -81) -> (-1, -81)
  line L1 (-1, -81) -> (-1, 1)
  line L2 (-1, 1) -> (161, 1)
  line L3 (161, 1) -> (161, -81)
  line L4 (2, -88) -> (158, -88)
  arc A0 (158, -88) -> (168, -78) centre (158, -78) ccw
  line L5 (168, -78) -> (168, -2)
  arc A1 (168, -2) -> (158, 8) centre (158, -2) ccw
  line L6 (158, 8) -> (2, 8)
  arc A2 (2, 8) -> (-8, -2) centre (2, -2) ccw
  line L7 (-8, -2) -> (-8, -78)
  arc A3 (-8, -78) -> (2, -88) centre (2, -78) ccw
extrude "Extrude19" add sketch "Sketch15" along normal blind 7 separate body contours L0 L1 L2 L3 | L4 A0 L5 A1 L6 A2 L7 A3 makes body 6
combine "Combine2" operation add target body 5 tool bodies 6
sketch "Sketch16" plane through (0, 0, -4.64) normal (0, 0, 1) x (-1, 0, 0)
  arc A0 (-2, -88) -> (8, -78) centre (-2, -78) ccw
  line L0 (8, -78) -> (8, -2)
  arc A1 (8, -2) -> (-2, 8) centre (-2, -2) ccw
  line L1 (-2, 8) -> (-158, 8)
  arc A2 (-158, 8) -> (-168, -2) centre (-158, -2) ccw
  line L2 (-168, -2) -> (-168, -78)
  arc A3 (-168, -78) -> (-158, -88) centre (-158, -78) ccw
  line L3 (-158, -88) -> (-2, -88)
  line L4 (-75.0636, -8.4943) -> (-75.1065, -8.4943)
  line L5 (-75.1065, -8.4943) -> (-75.1065, -71.4943)
  line L6 (-75.1065, -71.4943) -> (-75.0655, -71.4943)
  arc A4 (-75.0655, -71.4943) -> (-72.1065, -74) centre (-72.1065, -71) ccw
  line L7 (-72.1065, -74) -> (-9, -74)
  arc A5 (-9, -74) -> (-6, -71) centre (-9, -71) ccw
  line L8 (-6, -71) -> (-6, -64)
  arc A6 (-3, -61) -> (-6, -64) centre (-3, -64) ccw
  line L9 (-3, -61) -> (0.5, -61)
  line L10 (0.5, -61) -> (0.5, -81)
  line L11 (0.5, -81) -> (-161, -81)
  line L12 (-161, -81) -> (-161, 0.5)
  line L13 (-161, 0.5) -> (0.5, 0.5)
  line L14 (0.5, 0.5) -> (0.5, -19)
  line L15 (0.5, -19) -> (-3, -19)
  arc A7 (-6, -16) -> (-3, -19) centre (-3, -16) ccw
  line L16 (-6, -16) -> (-6, -9)
  arc A8 (-6, -9) -> (-9, -6) centre (-9, -9) ccw
  line L17 (-9, -6) -> (-72.1065, -6)
  arc A9 (-72.1065, -6) -> (-75.0636, -8.4943) centre (-72.1065, -9) ccw
  line L18 (0.5, -81) -> (-161, -81)
  line L19 (-161, -81) -> (-161, 0.5)
  line L20 (-161, 0.5) -> (0.5, 0.5)
  line L21 (0.5, 0.5) -> (0.5, -81)
  line L22 (0.5, -61) -> (8, -61)
  line L23 (8, -61) -> (8, -18.999)
  line L24 (8, -18.999) -> (0.5, -18.999)
  line L25 (0.5, -18.999) -> (0.5, -61)
  line L26 (4.25, -18.999) -> (4.25, -61)
  line L27 (8.2113, -27.4995) -> (0.2887, -27.4995)
  line L28 (0.2887, -27.4995) -> (0.2887, -52.4995)
  line L29 (0.2887, -52.4995) -> (8.2113, -52.4995)
  line L30 (8.2113, -52.4995) -> (8.2113, -27.4995)
  line L31 (8.2113, -27.4995) -> (0.2887, -52.4995) construction
  line L32 (0.2887, -27.4995) -> (8.2113, -52.4995) construction
  point P0 (4.25, -39.9995)
  dimension "d89" = 25
  constraint horizontal L18
  constraint vertical L19
  constraint horizontal L20
  constraint vertical L21
  constraint coincident L12.end L13.start
  constraint coincident L10.end L11.start
  constraint horizontal L22
  constraint vertical L23
  constraint horizontal L24
  constraint vertical L25
  constraint coincident L0 L23.end
  constraint coincident L9.end L10.start
  constraint midpoint L24 L26.start
  constraint midpoint L22 L26.end
  constraint perpendicular L22 L26
  constraint horizontal L27
  constraint perpendicular L27 L28
  constraint parallel L27 L29
  constraint parallel L28 L30
  constraint coincident L31 P0
  constraint coincident L32 P0
  constraint midpoint L26 P0
  measures "d89" distance of L27.end L28.end
extrude "Extrude20" cut sketch "Sketch16" against normal blind 4 contours L4 L5 L6 A4 L7 A5 L8 A6 L9 L15 A7 L16 A8 L17 A9 L21 L25 L27 L28 L29 | L21 L25 L27 L28 L29 bodies 5
extrude "Extrude21" cut sketch "Sketch16" along normal blind 4.64 contours L0 L23 L26 L27 L29 | L21 L25 L26 L27 L29 bodies 3
fillet "Fillet1" radius 2 2 edges at (-4.5, 52.4995, 0) (-4.5, 27.4995, 0) on bodies 3
extrude "Extrude22" cut sketch "Sketch16" against normal blind 4 contours L0 L23 L26 L27 L29 | L21 L25 L26 L27 L29 bodies 5
fillet "Fillet2" radius 2 2 edges at (-4.25, 27.4995, -8.64) (-4.25, 52.4995, -8.64) on bodies 5
fillet "Fillet4" radius 2 8 edges at (80, -8, 12.36) (165.0711, -5.0711, 12.36) (168, 40, 12.36) (165.0711, 85.0711, 12.36) (80, 88, 12.36) (-5.0711, 85.0711, 12.36) (-8, 40, 12.36) (-5.0711, -5.0711, 12.36) on bodies 3
sketch "Sketch17" plane through (0, 0, -11.64) normal (0, 0, -1) x (1, 0, 0)
  arc A0 (-8, -78) -> (2, -88) centre (2, -78) ccw
  line L0 (2, -88) -> (158, -88)
  arc A1 (158, -88) -> (168, -78) centre (158, -78) ccw
  line L1 (168, -78) -> (168, -2)
  arc A2 (168, -2) -> (158, 8) centre (158, -2) ccw
  line L2 (158, 8) -> (2, 8)
  arc A3 (2, 8) -> (-8, -2) centre (2, -2) ccw
  line L3 (-8, -2) -> (-8, -78)
  line L4 (2, 8) -> (22, 8)
  line L5 (22, 8) -> (22, 5.5) construction
  circle A4 centre (22, 5.5) radius 1.5
  line L6 (158, 8) -> (138, 8) construction
  line L7 (138, 8) -> (138, 5.5) construction
  circle A5 centre (138, 5.5) radius 1.5
  line L8 (158, -88) -> (138, -88)
  line L9 (138, -88) -> (138, -85.5) construction
  line L10 (138, -85.5) -> (158, -85.5) construction
  line L11 (158, -85.5) -> (158, -88)
  circle A6 centre (138, -85.5) radius 1.5
  line L12 (2, -88) -> (22, -88) construction
  line L13 (22, -88) -> (22, -85.5) construction
  line L14 (22, -85.5) -> (2, -85.5) construction
  line L15 (2, -85.5) -> (2, -88) construction
  circle A7 centre (22, -85.5) radius 1.5
  line L16 (-8, -78) -> (-4.5, -78) construction
  line L17 (-4.5, -78) -> (-4.5, -68) construction
  line L18 (-4.5, -68) -> (-8, -68) construction
  line L19 (-8, -68) -> (-8, -78) construction
  circle A8 centre (-4.5, -68) radius 1.5
  line L20 (-8, -2) -> (-4.5, -2) construction
  line L21 (-4.5, -2) -> (-4.5, -12) construction
  line L22 (-4.5, -12) -> (-8, -12) construction
  line L23 (-8, -12) -> (-8, -2) construction
  circle A9 centre (-4.5, -12) radius 1.5
  line L24 (168, -78) -> (164.5, -78) construction
  line L25 (164.5, -78) -> (164.5, -68) construction
  line L26 (164.5, -68) -> (168, -68) construction
  line L27 (168, -68) -> (168, -78) construction
  circle A10 centre (164.5, -68) radius 1.5
  line L28 (168, -2) -> (164.5, -2) construction
  line L29 (164.5, -2) -> (164.5, -12) construction
  line L30 (164.5, -12) -> (168, -12) construction
  line L31 (168, -12) -> (168, -2) construction
  circle A11 centre (164.5, -12) radius 1.5
  circle A12 centre (164.5, -12) radius 2.25
  circle A13 centre (164.5, -68) radius 2.25
  circle A14 centre (-4.5, -68) radius 2.25
  circle A15 centre (-4.5, -12) radius 2.25
  dimension "d102" = 20
  dimension "d103" = 2.5
  dimension "d104" = 3
  dimension "d105" = 20
  dimension "d106" = 2.5
  dimension "d107" = 3
  dimension "d108" = 20
  dimension "d109" = 2.5
  dimension "d110" = 3
  dimension "d111" = 20
  dimension "d112" = 2.5
  dimension "d113" = 3
  dimension "d114" = 3.5
  dimension "d115" = 10
  dimension "d116" = 3
  dimension "d117" = 3.5
  dimension "d118" = 10
  dimension "d119" = 3
  dimension "d120" = 3.5
  dimension "d121" = 10
  dimension "d122" = 3
  dimension "d123" = 3.5
  dimension "d124" = 10
  dimension "d125" = 3
  dimension "d126" = 4.5
  dimension "d127" = 4.5
  dimension "d128" = 4.5
  dimension "d129" = 4.5
  constraint coincident L2.end A3.start
  constraint parallel L2 L4
  constraint perpendicular L4 L5
  constraint coincident L5.end A4.centre
  constraint coincident A2.end L2.start
  constraint parallel L2 L6
  constraint vertical L7
  constraint coincident L7.end A5.centre
  constraint horizontal L8
  constraint vertical L9
  constraint horizontal L10
  constraint vertical L11
  constraint coincident L0.end A1.start
  constraint coincident L9.end L10.start
  constraint horizontal L12
  constraint vertical L13
  constraint horizontal L14
  constraint vertical L15
  constraint coincident A0.end L0.start
  constraint coincident L13.end L14.start
  constraint horizontal L16
  constraint vertical L17
  constraint horizontal L18
  constraint vertical L19
  constraint coincident A0.start L3.end
  constraint coincident L17.end L18.start
  constraint horizontal L20
  constraint vertical L21
  constraint horizontal L22
  constraint vertical L23
  constraint coincident A3.end L3.start
  constraint coincident L21.end L22.start
  constraint horizontal L24
  constraint vertical L25
  constraint horizontal L26
  constraint vertical L27
  constraint coincident A1.end L1.start
  constraint coincident L25.end L26.start
  constraint horizontal L28
  constraint vertical L29
  constraint horizontal L30
  constraint vertical L31
  constraint coincident L1.end A2.start
  constraint coincident L29.end L30.start
  constraint concentric A11 A12
  constraint concentric A10 A13
  constraint concentric A8 A14
  constraint concentric A9 A15
  measures "d102" distance of L2.end L4.end
  measures "d103" distance of L4.end L5.end
  measures "d104" diameter of A4
  measures "d105" distance of A2.end L6.end
  measures "d106" distance of L6.end L7.end
  measures "d107" diameter of A5
  measures "d108" distance of L0.end L8.end
  measures "d109" distance of L0.end L10.end
  measures "d110" diameter of A6
  measures "d111" distance of A0.end L12.end
  measures "d112" distance of A0.end L14.end
  measures "d113" diameter of A7
  measures "d114" distance of A0.start L16.end
  measures "d115" distance of A0.start L18.end
  measures "d116" diameter of A8
  measures "d117" distance of A3.end L20.end
  measures "d118" distance of A3.end L22.end
  measures "d119" diameter of A9
  measures "d120" distance of A1.end L24.end
  measures "d121" distance of A1.end L26.end
  measures "d122" diameter of A10
  measures "d123" distance of L1.end L28.end
  measures "d124" distance of L1.end L30.end
  measures "d125" diameter of A11
  measures "d126" diameter of A12
  measures "d127" diameter of A13
  measures "d128" diameter of A14
  measures "d129" diameter of A15
extrude "Extrude23" cut sketch "Sketch17" against normal blind 7 contours A8 | A9 | A10 | A11 | A12 | A13 | A14 | A15 bodies 5
extrude "Extrude24" cut sketch "Sketch17" against normal blind 15 contours A8 | A9 | A10 | A11 bodies 3
named bodies: "offsetter", "diffuser", "front case", "back case"
